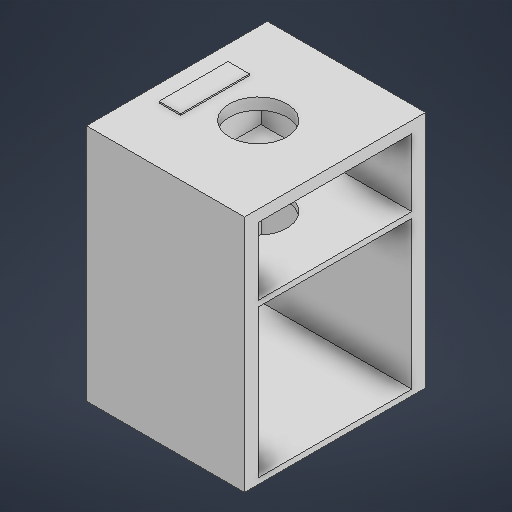
# Autodesk Inventor part: Table
Saved by Autodesk Inventor 2025.1 (Build 291241020, 241B)
## iProperties
Created: 2024-07-29
Part Number: Table
Material: Generic
Document SubType Name: Modeling
Designer: balmo
Density: 1 g/cm^3
Appearance: Default
Author: balmo
Autodesk Inventor part; units mm, degrees
ref_plane "YZ Plane" through (0, 0, 0) normal (1, 0, 0) x (0, 1, 0)
ref_plane "XZ Plane" through (0, 0, 0) normal (0, 1, 0) x (-1, 0, 0)
ref_plane "XY Plane" through (0, 0, 0) normal (0, 0, 1) x (1, 0, 0)
sketch "Sketch1" plane through (0, 0, 0) normal (0, 1, 0) x (-1, 0, 0)
  line L0 (0, 0) -> (349.25, 0)
  line L1 (349.25, 0) -> (349.25, -400.05)
  line L2 (349.25, -400.05) -> (0, -400.05)
  line L3 (0, -400.05) -> (0, 0)
  dimension "d0" = 400.05
  dimension "d1" = 349.25
  constraints: 8 end point, 2 parallel, 1 horizontal, 1 perpendicular
  measures "d0" distance of L2.end L0.start
  measures "d1" distance of L1.end L2.end
extrude "Extrusion1" add sketch "Sketch1" along normal blind 352.425
sketch "Sketch2" plane through (0, 0, 0) normal (1, 0, 0) x (0, 0, -1)
  line L0 (30.1625, 339.725) -> (369.8875, 339.725)
  line L1 (369.8875, 339.725) -> (369.8875, 12.7)
  line L2 (369.8875, 12.7) -> (30.1625, 12.7)
  line L3 (30.1625, 12.7) -> (30.1625, 339.725)
  line L4 (0, 0) -> (400.05, 0) projected
  line L5 (0, 352.425) -> (400.05, 352.425) projected
  line L6 (0, 0) -> (0, 352.425) projected
  line L7 (400.05, 0) -> (400.05, 352.425) projected
  dimension "d4" = 12.7
  dimension "d5" = 12.7
  dimension "d6" = 339.725
  dimension "d7" = 30.1625
  dimension "d8" = 30.1625
  constraints: 8 end point, 2 parallel, 1 horizontal, 1 perpendicular
  measures "d4" distance between parallel lines of L2 L4
  measures "d5" distance between parallel lines of L5 L0
  measures "d6" distance between parallel lines of L1 L3
  measures "d7" distance between parallel lines of L6 L3
  measures "d8" distance between parallel lines of L7 L1
extrude "Extrusion2" cut sketch "Sketch2" against normal blind 333.375 contours L0 L1 L2 L3
sketch "Sketch3" plane through (0, 352.425, 0) normal (0, 1, 0) x (1, 0, 0)
  line L0 (0, 400.05) -> (-349.25, 400.05) projected
  line L1 (-349.25, 400.05) -> (-349.25, 0) projected
  line L2 (-349.25, 0) -> (0, 0) projected
  line L3 (0, 0) -> (0, 400.05) projected
extrude "Extrusion3" add sketch "Sketch3" along normal blind 174.625
sketch "Sketch4" plane through (0, 0, 0) normal (1, 0, 0) x (0, 0, -1)
  line L0 (369.8875, 339.725) -> (369.8875, 12.7) projected
  line L1 (369.8875, 12.7) -> (30.1625, 12.7) projected
  line L2 (30.1625, 12.7) -> (30.1625, 339.725) projected
  line L3 (30.1625, 339.725) -> (369.8875, 339.725) projected
  line L4 (0, 0) -> (400.05, 0) projected
  line L5 (400.05, 0) -> (400.05, 527.05) projected
  line L6 (0, 527.05) -> (400.05, 527.05) projected
  line L7 (0, 0) -> (0, 527.05) projected
  line L8 (30.1625, 501.65) -> (369.8875, 501.65)
  line L9 (369.8875, 501.65) -> (369.8875, 352.425)
  line L10 (369.8875, 352.425) -> (30.1625, 352.425)
  line L11 (30.1625, 352.425) -> (30.1625, 501.65)
  point P0 (200.025, 501.65)
  dimension "d13" = 12.7
  dimension "d14" = 25.4
  constraints: 8 end point, 2 parallel, 1 horizontal, 1 midpoint, 1 perpendicular
  measures "d13" distance between parallel lines of L10 L3
  measures "d14" distance from line of L6 point (200.025, 501.65)
extrude "Extrusion4" cut sketch "Sketch4" against normal blind 333.375 contours L8 L9 L10 L11
sketch "Sketch5" plane through (0, 527.05, 0) normal (0, 1, 0) x (1, 0, 0)
  line L0 (-349.25, 400.05) -> (-349.25, 0) projected
  line L1 (-349.25, 0) -> (0, 0) projected
  line L2 (0, 0) -> (0, 400.05) projected
  line L3 (0, 400.05) -> (-349.25, 400.05) projected
  circle A0 centre (-169.8625, 200.025) radius 63.5
  line L4 (-106.3625, 200.025) -> (0, 200.025) construction
  dimension "d17" = 127
  dimension "d20" = 106.3625
  constraints: 2 end point, 1 horizontal alignment, 1 midpoint, 2 other
  measures "d20" distance of L4.start L4.end
extrude "Extrusion5" cut sketch "Sketch5" against normal blind 193.675 contours A0
sketch "Sketch6" plane through (0, 527.05, 0) normal (0, 1, 0) x (1, 0, 0)
  line L0 (-312.7375, 123.825) -> (-265.1125, 123.825)
  line L1 (-265.1125, 123.825) -> (-265.1125, 276.225)
  line L2 (-265.1125, 276.225) -> (-312.7375, 276.225)
  line L3 (-312.7375, 276.225) -> (-312.7375, 123.825)
  line L4 (-349.25, 400.05) -> (-349.25, 0) projected
  line L5 (-349.25, 0) -> (0, 0) projected
  line L6 (0, 400.05) -> (-349.25, 400.05) projected
  line L7 (0, 0) -> (0, 400.05) projected
  circle A0 centre (-169.8625, 200.025) radius 63.5 projected
  line L8 (-233.3625, 200.025) -> (-265.1125, 200.025)
  dimension "d23" = 152.4
  dimension "d24" = 47.625
  dimension "d26" = 123.825
  dimension "d27" = 123.825
  dimension "d32" = 265.1125
  constraints: 10 end point, 2 parallel, 1 horizontal, 1 horizontal alignment, 1 midpoint, 1 perpendicular, 1 other
  measures "d23" distance of L0.end L1.end
  measures "d24" distance of L0.start L0.end
  measures "d26" distance between parallel lines of L5 L0
  measures "d27" distance between parallel lines of L6 L2
  measures "d32" distance between parallel lines of L7 L1
extrude "Extrusion6" add sketch "Sketch6" along normal blind 3.175 and the other way blind 38.1 contours L3 L2 L1 L0
body "Solid1"
